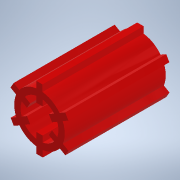
# Autodesk Inventor part: outerShaft
Saved by Autodesk Inventor 2021 (Build 250183000, 183)
## iProperties
Created: 2020-06-26
Part Number: outerShaft
Material: PET Plastic
Document SubType Name: Modeling
Designer: robst
Density: 1.541 g/cm^3
Appearance: Red
Author: robst
Autodesk Inventor part; units mm, degrees
ref_plane "YZ Plane" through (0, 0, 0) normal (1, 0, 0) x (0, 1, 0)
ref_plane "XZ Plane" through (0, 0, 0) normal (0, 1, 0) x (-1, 0, 0)
ref_plane "XY Plane" through (0, 0, 0) normal (0, 0, 1) x (1, 0, 0)
sketch "Sketch1" plane through (0, 0, 0) normal (0, 0, 1) x (1, 0, 0)
  circle A0 centre (0, 0) radius 12.7
  line L0 (-0.074, 12.6998) -> (-0.074, 15.8748) construction
  line L1 (-0.074, 15.8748) -> (1.5135, 15.8748)
  line L2 (1.5135, 15.8748) -> (1.5135, 12.6095)
  line L3 (-0.074, 15.8748) -> (-1.6615, 15.8748)
  line L4 (-1.6615, 15.8748) -> (-1.6615, 12.5909)
  line L5 (-14.5787, 6.4985) -> (-11.7347, 4.8566)
  line L6 (-13.7849, 7.8733) -> (-14.5787, 6.4985)
  line L7 (-13.7849, 7.8733) -> (-12.9912, 9.2482)
  line L8 (-12.9912, 9.2482) -> (-10.1634, 7.6155)
  line L9 (-12.9172, -9.3763) -> (-10.0733, -7.7343)
  line L10 (-13.711, -8.0014) -> (-12.9172, -9.3763)
  line L11 (-13.711, -8.0014) -> (-14.5047, -6.6266)
  line L12 (-14.5047, -6.6266) -> (-11.6769, -4.994)
  line L13 (1.6615, -15.8748) -> (1.6615, -12.5909)
  line L14 (0.074, -15.8748) -> (1.6615, -15.8748)
  line L15 (0.074, -15.8748) -> (-1.5135, -15.8748)
  line L16 (-1.5135, -15.8748) -> (-1.5135, -12.6095)
  line L17 (14.5787, -6.4985) -> (11.7347, -4.8566)
  line L18 (13.7849, -7.8733) -> (14.5787, -6.4985)
  line L19 (13.7849, -7.8733) -> (12.9912, -9.2482)
  line L20 (12.9912, -9.2482) -> (10.1634, -7.6155)
  line L21 (12.9172, 9.3763) -> (10.0733, 7.7343)
  line L22 (13.711, 8.0014) -> (12.9172, 9.3763)
  line L23 (13.711, 8.0014) -> (14.5047, 6.6266)
  line L24 (14.5047, 6.6266) -> (11.6769, 4.994)
  line L25 (0, 0) -> (0, 9.525) construction
  line L26 (0, 6.35) -> (1.5875, 6.35)
  line L27 (1.5875, 6.35) -> (1.5875, 9.3918)
  line L28 (0, 6.35) -> (-1.5875, 6.35)
  line L29 (-1.5875, 6.35) -> (-1.5875, 9.3918)
  line L30 (-6.293, 1.8002) -> (-8.9273, 3.3211)
  line L31 (-5.4993, 3.175) -> (-6.293, 1.8002)
  line L32 (-5.4993, 3.175) -> (-4.7055, 4.5498)
  line L33 (-4.7055, 4.5498) -> (-7.3398, 6.0707)
  line L34 (-4.7055, -4.5498) -> (-7.3398, -6.0707)
  line L35 (-5.4993, -3.175) -> (-4.7055, -4.5498)
  line L36 (-5.4993, -3.175) -> (-6.293, -1.8002)
  line L37 (-6.293, -1.8002) -> (-8.9273, -3.3211)
  line L38 (1.5875, -6.35) -> (1.5875, -9.3918)
  line L39 (0, -6.35) -> (1.5875, -6.35)
  line L40 (0, -6.35) -> (-1.5875, -6.35)
  line L41 (-1.5875, -6.35) -> (-1.5875, -9.3918)
  line L42 (6.293, -1.8002) -> (8.9273, -3.3211)
  line L43 (5.4993, -3.175) -> (6.293, -1.8002)
  line L44 (5.4993, -3.175) -> (4.7055, -4.5498)
  line L45 (4.7055, -4.5498) -> (7.3398, -6.0707)
  line L46 (4.7055, 4.5498) -> (7.3398, 6.0707)
  line L47 (5.4993, 3.175) -> (4.7055, 4.5498)
  line L48 (5.4993, 3.175) -> (6.293, 1.8002)
  line L49 (6.293, 1.8002) -> (8.9273, 3.3211)
  arc A1 (7.3398, 6.0707) -> (1.5875, 9.3918) centre (0, 0) ccw
  arc A2 (8.9273, -3.3211) -> (8.9273, 3.3211) centre (0, 0) ccw
  arc A3 (1.5875, -9.3918) -> (7.3398, -6.0707) centre (0, 0) ccw
  arc A4 (-7.3398, -6.0707) -> (-1.5875, -9.3918) centre (0, 0) ccw
  arc A5 (-1.5875, 9.3918) -> (-7.3398, 6.0707) centre (0, 0) ccw
  arc A6 (-8.9273, 3.3211) -> (-8.9273, -3.3211) centre (0, 0) ccw
  dimension "outerDiameter" = 25.4
  dimension "splineHeight" = 3.175
  dimension "splineWidth" = 3.175
  dimension "d16" = 360
  dimension "d20" = 3.175
  dimension "d21" = 3.175
  dimension "d24" = 360
  constraints: 100 end point, 15 point on circle, 7 centre point, 4 horizontal, 4 vertical, 2 coincident, 2 equal length, 2 perpendicular, 1 point on line, 110 other
  measures "outerDiameter" diameter of A0
  measures "splineHeight" distance of L0.start L0.end
  measures "splineWidth" distance between parallel lines of L4 L2
  measures "d20" distance from line of L26 L25.end
  measures "d21" distance between parallel lines of L29 L27
extrude "Extrusion4" add sketch "Sketch1" against normal blind 50.8
equation "\"d20\" = splineHeight"
equation "\"d21\" = splineWidth"
body "Solid4"
